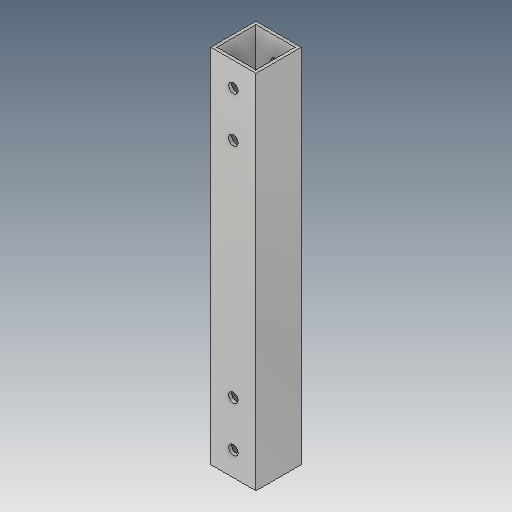
# Autodesk Inventor part: PitchSquarePipe
Saved by Autodesk Inventor 2019.4 (Build 234330000, 330)
## iProperties
Created: 2019-06-11
Part Number: PitchSquarePipe
Material: アルミニウム 5005-H12
Document SubType Name: Modeling
Designer: AzLIer
Density: 2.7 g/cm^3
Appearance: アルミニウム - つや出し
Mass: 17.9703 g
Surface Area: 135.037 cm^2
Volume: 6.65566 cm^3
Author: AzLIer
Autodesk Inventor part; units mm, degrees
ref_plane "YZ Plane" through (0, 0, 0) normal (1, 0, 0) x (0, 1, 0)
ref_plane "XZ Plane" through (0, 0, 0) normal (0, 1, 0) x (-1, 0, 0)
ref_plane "XY Plane" through (0, 0, 0) normal (0, 0, 1) x (1, 0, 0)
sketch "スケッチ1" plane through (0, 0, 0) normal (0, 1, 0) x (-1, 0, 0)
  line L0 (7.5, -7.5) -> (-7.5, -7.5)
  line L1 (-7.5, -7.5) -> (-7.5, 7.5)
  line L2 (-7.5, 7.5) -> (7.5, 7.5)
  line L3 (7.5, 7.5) -> (7.5, -7.5)
  line L4 (7.5, -7.5) -> (-7.5, 7.5) construction
  line L5 (-7.5, -7.5) -> (7.5, 7.5) construction
  point P0 (0, 0)
  dimension "d0" = 15
  dimension "d1" = 15
  constraints: 12 end point, 2 midpoint, 2 parallel, 1 horizontal, 1 perpendicular
  measures "d0" distance of L1.end L2.end
  measures "d1" distance of L0.end L1.end
extrude "押し出し1" add sketch "スケッチ1" along normal blind 120
shell "シェル1" thickness 1 removed faces 2 at (-2.5, 0, -2.5) at (-2.5, 120, -2.5)
sketch "スケッチ2" plane through (-7.5, 0, 7.5) normal (0, 0, 1) x (1, 0, 0)
  line L0 (15, 0) -> (0, 0) projected
  line L1 (0, 120) -> (15, 120) projected
  point P0 (7.5, 0)
  point P1 (7.5, 8)
  point P2 (7.5, 23)
  point P3 (7.5, 0)
  point P4 (7.5, 112)
  point P5 (7.5, 97)
  point P6 (7.5, 120)
  dimension "d5" = 8
  dimension "d6" = 15
  dimension "d14" = 8
  dimension "d15" = 15
  constraints: 4 vertical alignment, 2 midpoint
  measures "d5" distance of point (7.5, 0) point (7.5, 8)
  measures "d6" distance of point (7.5, 23) point (7.5, 8)
  measures "d14" distance from line of L1 point (7.5, 112)
  measures "d15" distance of point (7.5, 112) point (7.5, 97)
hole "穴1" at (0, 8, 7.5) at (0, 23, 7.5) at (0, 112, 7.5) at (0, 97, 7.5) direction (0, 0, -1) diameter 3.2 end through all
